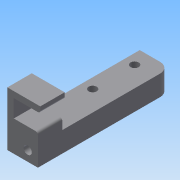
# Autodesk Inventor part: photoTransistorHolderLeft
Saved by Autodesk Inventor 2015 SP1 (Build 190203100, 203)
## iProperties
Created: 2015-06-25
Part Number: photoTransistorHolderLeft
Material: Generic
Document SubType Name: Modeling
Designer: Workstation
Density: 1 g/cm^3
Appearance: Default
Author: Workstation
Autodesk Inventor part; units mm, degrees
ref_plane "YZ Plane" through (0, 0, 0) normal (1, 0, 0) x (0, 1, 0)
ref_plane "XZ Plane" through (0, 0, 0) normal (0, 1, 0) x (-1, 0, 0)
sketch "Sketch1" plane through (0, 0, 0) normal (0, 1, 0) x (-1, 0, 0)
  line L0 (0, 0) -> (0, -41.275)
  line L1 (0, -41.275) -> (0, -36.5125)
  line L2 (0, -36.5125) -> (0, -23.4315)
  circle A0 centre (0, -36.5125) radius 1.27
  circle A1 centre (0, -23.4315) radius 1.27
  line L3 (0, -41.275) -> (3.175, -41.275)
  line L4 (3.175, -41.275) -> (3.175, 0)
  line L5 (3.175, 0) -> (0, 0)
  line L6 (0, -41.275) -> (-6.35, -41.275)
  line L7 (-6.35, -41.275) -> (-6.35, 0)
  line L8 (-6.35, 0) -> (0, 0)
  dimension "d0" = 41.275
  dimension "d1" = 4.7625
  dimension "d2" = 13.081
  dimension "d3" = 2.54
  dimension "d4" = 2.54
  dimension "d5" = 3.175
  dimension "d6" = 6.35
  constraints: 18 end point, 4 perpendicular, 4 point on line, 2 centre point, 2 coincident, 1 horizontal, 1 vertical
  measures "d0" distance of L0.start L0.end
  measures "d1" distance of L0.end L1.end
  measures "d2" distance of L1.end L2.end
  measures "d3" diameter of A0
  measures "d4" diameter of A1
  measures "d5" distance of L0.end L3.end
  measures "d6" distance of L0.end L6.end
extrude "Extrusion1" add sketch "Sketch1" along normal blind 6.35
extrude "Extrusion2" cut sketch "Sketch1" along normal blind 6.35 contours A1 L0 | L0 A1 | A0 L0 | L0 A0
sketch "Sketch3" plane through (-3.175, 0, 0) normal (0, 0, 1) x (1, 0, 0)
  line L0 (0, 0) -> (9.525, 0) projected
  line L1 (9.525, 0) -> (9.525, 6.35) projected
  line L2 (0, 6.35) -> (9.525, 6.35) projected
  line L3 (0, 0) -> (0, 6.35) projected
  circle A0 centre (6.35, 3.175) radius 1.27
  line L4 (6.35, 3.175) -> (2.0066, 3.175)
  line L5 (2.0066, 3.175) -> (2.0066, 0)
  line L6 (9.525, 0) -> (0, 0) projected
  line L7 (6.35, 3.175) -> (6.35, -8.6614)
  line L8 (2.0066, 0) -> (2.0066, -8.6614)
  line L9 (2.0066, -8.6614) -> (2.0066, -10.5664)
  line L10 (2.0066, -10.5664) -> (10.2616, -10.5664)
  line L11 (10.2616, -10.5664) -> (10.2616, -8.6614)
  line L12 (10.2616, -8.6614) -> (6.35, -8.6614)
  line L13 (0, 0) -> (0, -10.5664)
  line L14 (0, -10.5664) -> (2.0066, -10.5664)
  line L15 (0, 0) -> (2.0066, 0)
  line L16 (6.35, -8.6614) -> (2.0066, -8.6614)
  line L17 (2.0066, -8.6614) -> (2.0066, 0)
  line L18 (6.35, 3.175) -> (6.35, -3.175)
  line L19 (9.525, 0) -> (2.0066, 0)
  line L20 (2.0066, 0) -> (2.0066, -3.175)
  line L21 (2.0066, -3.175) -> (9.525, -3.175)
  line L22 (9.525, -3.175) -> (9.525, 0)
  point P0 (3.175, 0)
  dimension "d11" = 2.54
  dimension "d14" = 3.175
  dimension "d15" = 9.525
  dimension "d16" = 4.3434
  dimension "d17" = 11.8364
  dimension "d18" = 1.905
  dimension "d19" = 8.255
  dimension "d22" = 6.35
  constraints: 36 end point, 9 perpendicular, 5 point on line, 4 parallel, 2 horizontal, 1 centre point, 1 vertical
  measures "d11" diameter of A0
  measures "d14" distance from line of L4.start L1
  measures "d15" distance between parallel lines of L3 L1
  measures "d16" distance of L4.start L4.end
  measures "d17" distance of L4.start L7.end
  measures "d18" distance of L8.end L9.end
  measures "d19" distance of L9.end L10.end
  measures "d22" distance of L4.start L18.end
extrude "Extrusion3" cut sketch "Sketch3" against normal blind 8.89 contours L7 L4 A0 | A0 L4 L7
extrude "Extrusion4" add sketch "Sketch3" against normal blind 7.62 contours L0 L8 L9 L14 L13 | L9 L16 L12 L11 L10
extrude "Extrusion5" add sketch "Sketch3" against normal blind 7.62 contours L0 L7 L21 L8 | L0 L22 L21 L7
fillet "Fillet1" radius 3.175 1 edges at (6.35, 3.175, -41.275)
fillet "Fillet2" radius 0.762 2 edges at (6.35, -3.175, -3.81) (7.0866, -8.6614, -3.81)
ref_plane "Work Plane1" through (0, 3.175, 0) normal (0, -1, 0) x (1, 0, 0)
mirror "Mirror1" about plane through (0, 3.175, 0) normal (0, -1, 0) of "Extrusion4", "Fillet2", "Extrusion5"
sketch "Sketch4" plane through (6.35, 0, -7.62) normal (1, 0, 0) x (0, 0, -1)
  line L0 (33.655, 0) -> (0, 0) projected
  line L1 (3.7313, 0) -> (-10.4318, 0)
  line L2 (-10.4318, 0) -> (-10.4318, -14.3979)
  line L3 (-10.4318, -14.3979) -> (3.7313, -14.3979)
  line L4 (3.7313, -14.3979) -> (3.7313, 0)
  point P0 (-7.62, 0)
  constraints: 8 end point, 2 parallel, 1 horizontal, 1 perpendicular, 1 point on line
extrude "Extrusion6" cut sketch "Sketch4" along normal blind 25.4 and the other way blind 12.7
body "Solid1"
